Autodesk Fusion 360 part; units mm, degrees
(part 7 of 7)
  spline S1422 degree 3 poles (-1.1853, -0.2876) (-1.0066, -0.2781) (-0.8826, -0.272) (-0.7429, -0.2668) knots 0 0 0 0 1 1 1 1
  spline S1423 degree 3 poles (-0.7429, -0.2668) (-0.6718, -0.2642) (-0.592, -0.2599) (-0.5677, -0.2573) knots 0 0 0 0 1 1 1 1
  spline S1424 degree 3 poles (-0.5677, -0.2573) (-0.5226, -0.2529) (-0.5218, -0.2521) (-0.5218, -0.2234) knots 0 0 0 0 1 1 1 1
  spline S1425 degree 3 poles (-0.5218, -0.2234) (-0.5218, -0.187) (-0.5374, -0.1775) (-0.5911, -0.1801) knots 0 0 0 0 1 1 1 1
  spline S1426 degree 3 poles (-0.5911, -0.1801) (-0.6128, -0.1809) (-0.7161, -0.1844) (-0.821, -0.1879) knots 0 0 0 0 1 1 1 1
  spline S1427 degree 3 poles (-0.821, -0.1879) (-0.926, -0.1905) (-1.0812, -0.2) (-1.1662, -0.2078) knots 0 0 0 0 1 1 1 1
  line L171 (-1.1662, -0.2078) -> (-1.3206, -0.2226)
  line L172 (-1.3206, -0.2226) -> (-1.318, -0.2573)
  spline S1428 degree 3 poles (-1.318, -0.2573) (-1.3163, -0.2764) (-1.312, -0.292) (-1.3068, -0.2928) knots 0 0 0 0 1 1 1 1
  spline S1429 degree 3 poles (-1.3068, -0.2928) (-1.3024, -0.2937) (-1.2478, -0.292) (-1.1853, -0.2876) knots 0 0 0 0 1 1 1 1
  spline S1430 degree 3 poles (1.9157, 6.4826) (2.0614, 6.5095) (2.1889, 6.5546) (2.1976, 6.5823) knots 0 0 0 0 1 1 1 1
  spline S1431 degree 3 poles (2.1976, 6.5823) (2.2054, 6.6075) (2.1941, 6.6335) (2.1751, 6.6335) knots 0 0 0 0 1 1 1 1
  spline S1432 degree 3 poles (2.1751, 6.6335) (2.1655, 6.6335) (2.1178, 6.6214) (2.0692, 6.6066) knots 0 0 0 0 1 1 1 1
  spline S1433 degree 3 poles (2.0692, 6.6066) (1.9938, 6.5832) (1.9634, 6.5789) (1.8619, 6.5745) knots 0 0 0 0 1 1 1 1
  spline S1434 degree 3 poles (1.8619, 6.5745) (1.757, 6.5711) (1.7379, 6.5728) (1.6867, 6.5901) knots 0 0 0 0 1 1 1 1
  spline S1435 degree 3 poles (1.6867, 6.5901) (1.6164, 6.6136) (1.5349, 6.6665) (1.4959, 6.7142) knots 0 0 0 0 1 1 1 1
  spline S1436 degree 3 poles (1.4959, 6.7142) (1.4803, 6.7341) (1.4508, 6.7827) (1.4308, 6.8226) knots 0 0 0 0 1 1 1 1
  spline S1437 degree 3 poles (1.4308, 6.8226) (1.4109, 6.8625) (1.3883, 6.8972) (1.3814, 6.8998) knots 0 0 0 0 1 1 1 1
  spline S1438 degree 3 poles (1.3814, 6.8998) (1.3744, 6.9024) (1.3579, 6.8998) (1.3458, 6.8946) knots 0 0 0 0 1 1 1 1
  spline S1439 degree 3 poles (1.3458, 6.8946) (1.318, 6.8816) (1.3215, 6.8651) (1.3736, 6.7593) knots 0 0 0 0 1 1 1 1
  spline S1440 degree 3 poles (1.3736, 6.7593) (1.4378, 6.6266) (1.5332, 6.5459) (1.6815, 6.4982) knots 0 0 0 0 1 1 1 1
  spline S1441 degree 3 poles (1.6815, 6.4982) (1.7205, 6.4852) (1.8749, 6.4748) (1.9157, 6.4826) knots 0 0 0 0 1 1 1 1
  spline S1442 degree 3 poles (-1.351, 6.4956) (-1.2573, 6.5182) (-1.1888, 6.5572) (-1.1159, 6.6292) knots 0 0 0 0 1 1 1 1
  spline S1443 degree 3 poles (-1.1159, 6.6292) (-1.0708, 6.6734) (-1.0457, 6.7072) (-1.0223, 6.755) knots 0 0 0 0 1 1 1 1
  spline S1444 degree 3 poles (-1.0223, 6.755) (-0.9719, 6.859) (-0.9711, 6.9024) (-1.0205, 6.9024) knots 0 0 0 0 1 1 1 1
  spline S1445 degree 3 poles (-1.0205, 6.9024) (-1.0361, 6.9024) (-1.0483, 6.8859) (-1.0856, 6.8157) knots 0 0 0 0 1 1 1 1
  spline S1446 degree 3 poles (-1.0856, 6.8157) (-1.1411, 6.7099) (-1.1957, 6.6552) (-1.2912, 6.6092) knots 0 0 0 0 1 1 1 1
  line L173 (-1.2912, 6.6092) -> (-1.3588, 6.5771)
  line L174 (-1.3588, 6.5771) -> (-1.4803, 6.5771)
  spline S1447 degree 3 poles (-1.4803, 6.5771) (-1.5904, 6.5771) (-1.613, 6.5797) (-1.7153, 6.6066) knots 0 0 0 0 1 1 1 1
  spline S1448 degree 3 poles (-1.7153, 6.6066) (-1.7778, 6.6231) (-1.8359, 6.6335) (-1.8437, 6.6309) knots 0 0 0 0 1 1 1 1
  spline S1449 degree 3 poles (-1.8437, 6.6309) (-1.8654, 6.6222) (-1.8602, 6.5849) (-1.8342, 6.565) knots 0 0 0 0 1 1 1 1
  spline S1450 degree 3 poles (-1.8342, 6.565) (-1.809, 6.5442) (-1.7058, 6.5112) (-1.6043, 6.4913) knots 0 0 0 0 1 1 1 1
  spline S1451 degree 3 poles (-1.6043, 6.4913) (-1.5167, 6.473) (-1.4351, 6.4748) (-1.351, 6.4956) knots 0 0 0 0 1 1 1 1
extrude "拉伸7" cut sketch "草图5" against normal blind 1 contours S478 S479 S480 S481 S482 S483 S484 S485 S486 S487 S488 S489 S490 S491 S492 S493 S494 S495 S496 S497 S498 S499 S500 S501 S502 S503 S504 S505 S506 S507 S508 S509 S510 S511 S512 S513 S514 S515 S516 S517 S518 S519 S520 S521 S522 S523 S524 S525 S526 S527 S528 S529 S530 S531 S532 S533 S534 S535 S536 S537 S538 S539 S540 L85 L86 S541 S542 S543 S544 S545 L87 L88 S546 S547 S548 S549 S550 S551 S552 S553 S554 S555 S556 S557 S558 S559 S560 L89 L90 S561 S562 S563 S564 S565 S566 S567 S568 S569 S570 S571 S572 S573 S574 S575 S576 S577 S578 S579 S580 S581 S582 S583 S584 S585 S586 S587 S588 S589 S590 S591 S592 S593 S594 S595 S596 S597 S598 S599 S600 S601 S602 S603 S604 S605 S606 S607 S608 S609 S610 S611 S612 S613 S614 S615 S616 S617 S618 S619 S620 S621 S622 S623 S624 S625 S626 S627 S628 S629 S630 S631 S632 S633 S634 S635 S636 S637 S638 S639 S640 S641 L91 L92 S642 S643 S644 S645 S646 L93 L94 S647 S648 S649 S650 S651 S652 S653 S654 S655 S656 S657 S658 S659 S660 S661 S662 S663 S664 S665 S666 S667 S668 S669 S670 S671 S672 S673 S674 S675 S676 S677 S678 S679 S680 S681 S682 S683 S684 S685 S686 S687 S688 S689 S690 S691 S692 S693 S694 S695 S696 S697 S698 S699 S700 S701 S702 S703 S704 S705 L95 L96 S706 S707 S708 S709 S710 S711 S712 S713 S714 S715 S716 S717 S718 S719 S720 S721 S722 S723 S724 S725 S726 S727 S728 S729 S730 S731 S732 S733 S734 S735 S736 S737 S738 S739 S740 S741 L97 L98 S742 S743 S744 S745 S746 S747 S748 S749 S750 S751 S752 S753 S754 S755 S756 S757 S758 S759 S760 S761 S762
extrude "拉伸8" cut sketch "草图5" against normal blind 1 contours S1410 S1411 S1412 S1413 S1414 S1415 S1416 S1417 S1418 S1419 S1420 S1421
extrude "拉伸9" cut 1 faces at (-0.1763, 2, 3.4987) along direction (0, -1, 0) blind 1
extrude "拉伸10" cut 13 faces at (0.0985, 2, 3.1181) (-0.1748, 2, 2.8964) (-0.4723, 2, 3.1355) (-0.2061, 2, 3.3481) (-0.0957, 2, 3.2575) (0.0245, 2, 3.2275) (0.4847, 2, 3.6702) (-0.0007, 2, 3.7008) (-0.3513, 2, 3.7134) (-0.2986, 2, 3.3839) (-0.8202, 2, 3.6347) (-0.4895, 2, 4.4075) (0.3992, 2, 4.7105) along direction (0, -1, 0) blind 1
